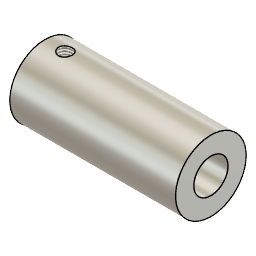
Corpo de prova (Autodesk Fusion 360 archive; units mm, degrees)
design "usinagem tarugo"
Autodesk Fusion 360 part; units mm, degrees
sketch "Esboço1" plane through (0, 0, 0) normal (0, 1, 0) x (1, 0, 0)
  line L0 (0, 0) -> (61, 0)
  dimension "d1" = 61
  constraint coincident L0.start origin
  constraint horizontal L0
  measures "d1" distance of L0.start L0.end
form "Forma1" [no effect]
cylinder "Cilindro primitivo1" add diameter 26 height 61 placed x (0, 0, -1) y (0, 1, 0) z (1, 0, 0) at (0, 0, 0) in component "Component"
hole "Furo1" at (61, 0, 0) direction (-1, 0, 0) diameter 12.6 depth 47 tip angle 180 in component "Component"
ref_plane "Plano de trabalho1" through (8.8555, 13, 0) normal (0, 1, 0) x (0, 0, -1)
sketch "Esboço4" plane through (0, 13, 0) normal (0, 1, 0) x (1, 0, 0)
  line L0 (0, 0) -> (7.5, 0)
  dimension "d12" = 7.5
  constraint coincident L0.start origin
  constraint horizontal L0
  measures "d12" distance of L0.start L0.end
hole "Furo3" at (7.5, 13, 0) direction (0, -1, 0) diameter 5.035 depth 13 tip angle 118 in component "Component"
thread "Rosca2" "ISO Metric profile 6.0 M6x1 M6x1 6H" thread offset 0 thread depth 7.4 in component "Component"
sketch "Esboço5" plane through (14, 0, 0) normal (1, 0, 0) x (0, 0, -1)
  circle A0 centre (0, 0) radius 6.3
  circle A1 centre (0, 0) radius 6.25
  dimension "d16" = 12.5
  constraint coincident A0.centre A1.centre
  measures "d16" diameter of A1
component "Component" placed x (1, 0, 0) y (0, 1, 0) z (0, 0, 1) at (0, 0, 0)
equation "d12 = 9 mm - 1.5 mm"
